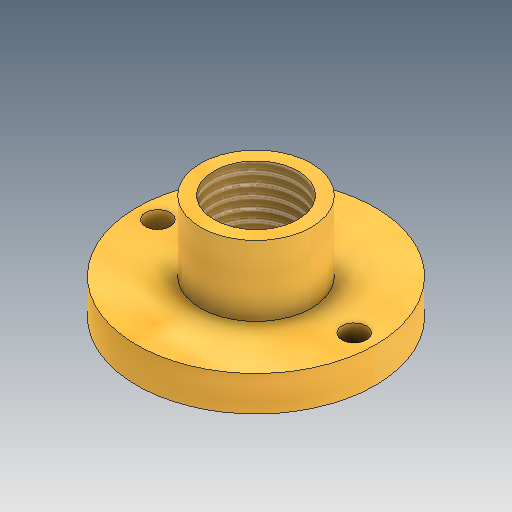
# Autodesk Inventor part: Tuerca de mesa
Saved by Autodesk Inventor 2020.3 (Build 243373000, 373)
## iProperties
Created: 2020-05-16
Part Number: Tuerca de mesa
Material: Brass, Soft Yellow
Document SubType Name: Modeling
Designer: Pipi
Density: 8.47 g/cm^3
Appearance: Bamboo
Mass: 38.654 g
Surface Area: 36.4817 cm^2
Volume: 4.56363 cm^3
Author: Pipi
Autodesk Inventor part; units mm, degrees
ref_plane "YZ Plane" through (0, 0, 0) normal (1, 0, 0) x (0, 1, 0)
ref_plane "XZ Plane" through (0, 0, 0) normal (0, 1, 0) x (-1, 0, 0)
ref_plane "XY Plane" through (0, 0, 0) normal (0, 0, 1) x (1, 0, 0)
sketch "Boceto1" plane through (0, 0, 0) normal (0, 1, 0) x (-1, 0, 0)
  circle A0 centre (10.3662, 9.9379) radius 6
  circle A1 centre (10.3662, 9.9379) radius 7.9
  circle A2 centre (10.3662, 9.9379) radius 17
  line L0 (18.2662, 9.9379) -> (22.6162, 9.9379)
  line L1 (2.4662, 9.9379) -> (-1.8838, 9.9379)
  line L2 (22.6162, 9.9379) -> (24.3662, 9.9379)
  line L3 (-1.8838, 9.9379) -> (-3.6338, 9.9379)
  circle A3 centre (24.3662, 9.9379) radius 1.75
  circle A4 centre (-3.6338, 9.9379) radius 1.75
  dimension "d0" = 12
  dimension "d1" = 15.8
  dimension "d35" = 34
  dimension "d40" = 14
  dimension "d41" = 14
  constraints: 8 end point, 4 coincident, 4 horizontal, 3 centre point, 2 horizontal alignment, 2 point on circle, 4 other
  measures "d0" diameter of A0
  measures "d1" diameter of A1
  measures "d35" diameter of A2
  measures "d40" distance of L2.end A0.centre
  measures "d41" distance of L3.end A0.centre
extrude "Extrusión6" add sketch "Boceto1" along normal blind 10 contours A1
extrude "Extrusión8" add sketch "Boceto1" against normal blind 5 contours A1 | A2
thread "Thread3" size "M12x1.5" class "6H" standard "ISO Metric profile" length 40
